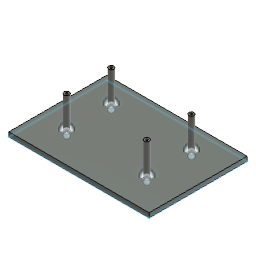
Display_support_V1 (Autodesk Fusion 360 design; units mm, degrees)
part number: 2026-04-17-10-27-17-697
Autodesk Fusion 360 part; units mm, degrees
sketch "Sketch1" plane through (0, 0, 0) normal (0, 1, 0) x (1, 0, 0)
  line L0 (-1.1736, -3.7554) -> (156.2264, -3.7554)
  line L1 (156.2264, -3.7554) -> (156.2264, -113.7554)
  line L2 (156.2264, -113.7554) -> (-1.1736, -113.7554)
  line L3 (-1.1736, -113.7554) -> (-1.1736, -3.7554)
  circle A0 centre (30, -30) radius 1.5
  circle A1 centre (120, -30) radius 1.5
  circle A2 centre (30, -80) radius 1.5
  circle A3 centre (120, -80) radius 1.5
  dimension "d1" = 157.4
  dimension "d2" = 110
  dimension "d3" = 3
  dimension "d4" = 3
  dimension "d5" = 3
  dimension "d6" = 3
  constraint horizontal L0
  constraint vertical L1
  constraint horizontal L2
  constraint vertical L3
  measures "d1" distance of L0.start L0.end
  measures "d2" distance of L0.start L2.end
  measures "d3" diameter of A0
  measures "d4" diameter of A1
  measures "d5" diameter of A2
  measures "d6" diameter of A3
extrude "Extrude1" add sketch "Sketch1" along normal blind 48.5 contours A0 makes body 1
extrude "Extrude2" add sketch "Sketch1" along normal blind 48.5 separate body contours A1 makes body 2
extrude "Extrude3" add sketch "Sketch1" along normal blind 28.5 separate body contours A2 makes body 3
extrude "Extrude4" add sketch "Sketch1" along normal blind 48.5 separate body contours A3 makes body 4
extrude "Extrude5" cut 1 faces at (30.1827, 28.5, 79.1007) along direction (0, -1, 0) blind 30 on bodies 3 bodies 3
extrude "Extrude6" add sketch "Sketch1" along normal blind 48.5 contours A2 bodies 3
extrude "Extrude7" add sketch "Sketch1" along normal blind 5 bodies 1 2 3 4
hole "Hole1" at (30, 48.5, 30) direction (0, -1, 0) diameter 2 depth 7 tip angle 180 bodies 1
hole "Hole2" at (30, 48.5, 80) direction (0, -1, 0) diameter 2 depth 7 tip angle 180 bodies 1
hole "Hole3" at (120, 48.5, 30) direction (0, -1, 0) diameter 2 depth 7 tip angle 180 bodies 1
hole "Hole4" at (120, 48.5, 80) direction (0, -1, 0) diameter 2 depth 7 tip angle 180 bodies 1
sketch "Sketch3" plane through (0, 5, 0) normal (0, 1, 0) x (-1, 0, 0)
  circle A0 centre (-120, 30) radius 1.5
  circle A1 centre (-30, 80) radius 1.5
  circle A2 centre (-30, 30) radius 1.5
  circle A3 centre (-120, 80) radius 1.5
  line L0 (1.1736, 113.7554) -> (-156.2264, 113.7554)
  line L1 (-156.2264, 113.7554) -> (-156.2264, 3.7554)
  line L2 (-156.2264, 3.7554) -> (1.1736, 3.7554)
  line L3 (1.1736, 3.7554) -> (1.1736, 113.7554)
  circle A4 centre (-30, 30) radius 3
  circle A5 centre (-120, 30) radius 3
  circle A6 centre (-120, 80) radius 3
  circle A7 centre (-30, 80) radius 3
  dimension "d33" = 6
  dimension "d34" = 6
  dimension "d35" = 6
  dimension "d36" = 6
  constraint concentric A2 A4
  constraint concentric A0 A5
  constraint concentric A3 A6
  constraint concentric A1 A7
  measures "d33" diameter of A4
  measures "d34" diameter of A5
  measures "d35" diameter of A6
  measures "d36" diameter of A7
extrude "Extrude8" add sketch "Sketch3" along normal blind 10 contours A6 bodies 1
delete_face "DeleteFace1" 1 faces at (121.4925, 26.1667, 79.8506) on bodies 1
extrude "Extrude9" add 1 faces at (118.5994, 15, 79.7052) along direction (0, 1, 0) blind 2 on bodies 1 bodies 1
extrude "Extrude10" add sketch "Sketch3" along normal blind 12 contours A5 bodies 1
extrude "Extrude11" add sketch "Sketch3" along normal blind 12 contours A4 bodies 1
extrude "Extrude12" add sketch "Sketch3" along normal blind 12 contours A7 bodies 1
delete_face "DeleteFace2" 1 faces at (31.4925, 27.5, 80.1494) on bodies 1
delete_face "DeleteFace3" 1 faces at (31.4925, 27.5, 30.1494) on bodies 1
delete_face "DeleteFace4" 1 faces at (121.4925, 27.5, 29.8506) on bodies 1
hole "Hole5" at (120, 17, 80) direction (0, -1, 0) diameter 2.1 depth 7 tip angle 180 bodies 1
hole "Hole6" at (30, 17, 80) direction (0, -1, 0) diameter 2.1 depth 7 tip angle 180 bodies 1
hole "Hole7" at (30, 17, 30) direction (0, -1, 0) diameter 2.1 depth 7 tip angle 180 bodies 1
hole "Hole8" at (120, 17, 30) direction (0, -1, 0) diameter 2.1 depth 7 tip angle 180 bodies 1
extrude "Extrude13" add 1 faces at (27.6621, 17, 29.8248) along direction (0, 1, 0) blind 24 on bodies 1 bodies 1
extrude "Extrude14" add 1 faces at (32.0303, 17, 81.1722) along direction (0, 1, 0) blind 24 on bodies 1 bodies 1
extrude "Extrude15" add 1 faces at (119.309, 17, 82.2403) along direction (0, 1, 0) blind 24 on bodies 1 bodies 1
extrude "Extrude16" add 1 faces at (120.691, 17, 27.7597) along direction (0, 1, 0) blind 24 on bodies 1 bodies 1
